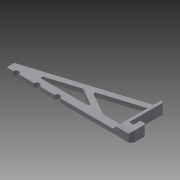
# Autodesk Inventor part: SpoolHandle2
Saved by Autodesk Inventor 2014 (Build 180170000, 170)
## iProperties
Created: 2014-04-03
Part Number: SpoolHandle2
Material: Generic
Document SubType Name: Modeling
Designer: Krzysiek
Density: 1 g/cm^3
Appearance: Default
Author: Krzysiek
Autodesk Inventor part; units mm, degrees
ref_plane "YZ Plane" through (0, 0, 0) normal (1, 0, 0) x (0, 1, 0)
ref_plane "XZ Plane" through (0, 0, 0) normal (0, 1, 0) x (-1, 0, 0)
ref_plane "XY Plane" through (0, 0, 0) normal (0, 0, 1) x (1, 0, 0)
sketch "Sketch1" plane through (0, 0, 0) normal (0, 0, 1) x (1, 0, 0)
  line L0 (0, 0) -> (0, -10)
  line L1 (0, -10) -> (8, -10)
  line L2 (8, -10) -> (8, 11)
  line L3 (-174, 11) -> (-174, 0)
  line L4 (-6.5, -50) -> (-6.5, 0)
  line L5 (-14.5, 0) -> (-14.5, -41.6161)
  line L6 (-80.6593, -20.8766) -> (-44.5, 0)
  line L7 (-44.5, 0) -> (-14.5, 0)
  line L8 (-91.0289, -17.6259) -> (-60.5, 0)
  line L9 (-60.5, 0) -> (-147.2555, 0)
  line L10 (-147.2555, 0) -> (-91.0289, -17.6259)
  line L11 (-6.5, 0) -> (0, 0)
  line L12 (-80.6593, -20.8766) -> (-14.5, -41.6161)
  arc A0 (-164, 11) -> (-156, 11) centre (-160, 11) ccw
  arc A1 (-134, 11) -> (-126, 11) centre (-130, 11) ccw
  arc A2 (-104, 11) -> (-96, 11) centre (-100, 11) ccw
  line L13 (-164, 11) -> (-174, 11)
  line L14 (-134, 11) -> (-156, 11)
  line L15 (8, 11) -> (-96, 11)
  line L16 (-104, 11) -> (-126, 11)
  line L17 (-174, 0) -> (-14.5, -50)
  line L18 (-14.5, -50) -> (-6.5, -50)
  line L19 (-164, 11) -> (-96, 11) construction
  dimension "d0" = 8
  dimension "d1" = 10
  dimension "d2" = 6.5
  dimension "d3" = 182
  dimension "d4" = 11
  dimension "d6" = 8
  dimension "d7" = 50
  dimension "d8" = 30
  dimension "d10" = 8
  dimension "d11" = 30
  dimension "d12" = 8
  dimension "d13" = 160
  dimension "d14" = 30
  dimension "d15" = 30
  dimension "d16" = 8
  dimension "d17" = 8
  constraints: 40 end point, 11 parallel, 7 collinear, 6 point on circle, 3 centre point, 2 equal radius, 2 horizontal, 2 perpendicular, 2 point on line, 1 horizontal alignment, 1 midpoint, 1 vertical
  measures "d0" distance of L0.end L1.end
  measures "d1" distance of L0.start L0.end
  measures "d2" distance of L4.end L0.start
  measures "d3" distance of L2.end L3.start
  measures "d4" distance of L3.start L3.end
  measures "d6" distance between parallel lines of L4 L5
  measures "d7" distance of L4.start L4.end
  measures "d8" distance of L6.end L5.start
  measures "d10" distance between parallel lines of L6 L8
  measures "d11" angle of L8 L9
  measures "d12" diameter of A0
  measures "d13" horizontal distance of A0.centre L0.start
  measures "d14" distance of A1.centre A0.centre
  measures "d15" distance of A2.centre A1.centre
  measures "d16" distance between parallel lines of L17 L12
  measures "d17" distance of L17.end L4.start
extrude "Extrusion1" add sketch "Sketch1" along normal blind 15
sketch "Sketch2" plane through (0, 0, 15) normal (0, 0, 1) x (1, 0, 0)
  line L0 (-174.5, 11) -> (-14.5, 11)
  line L1 (-14.5, 11) -> (-14.5, -59)
  line L2 (-14.5, -59) -> (-174.5, -59)
  line L3 (-174.5, -59) -> (-174.5, 11)
  line L4 (-6.5, 0) -> (0, 0) projected
  line L5 (-14.5, 0) -> (-14.5, -41.6161) projected
  line L6 (8, 11) -> (-96, 11) projected
  dimension "d20" = 70
  dimension "d21" = 160
  constraints: 8 end point, 2 collinear, 2 parallel, 1 horizontal, 1 perpendicular
  measures "d20" distance of L0.end L1.end
  measures "d21" distance of L0.start L0.end
extrude "Extrusion2" cut sketch "Sketch2" against normal blind 9
chamfer "Chamfer1" distance 4 angle 45 1 edges at (8, 11, 7.5)
chamfer "Chamfer2" distance 4 angle 45 1 edges at (-5.25, 11, 15)
chamfer "Chamfer3" distance 2 angle 45 1 edges at (8, -10, 7.5)
chamfer "Chamfer4" distance 4 angle 45 1 edges at (-14.5, -21.5, 15)
chamfer "Chamfer5" distance 5 angle 45 2 edges at (-14.5, -45.8081, 6) (-14.5, 5.5, 6)
fillet "Fillet1" radius 2 1 edges at (-147.2555, 0, 3)
fillet "Fillet2" radius 2 8 edges at (-80.6593, -20.8766, 3) (-44.5, 0, 3) (-60.5, 0, 3) (-91.0289, -17.6259, 3) (-14.5, 0, 8.5) (-14.5, 0, 3) (-14.5, -41.6161, 8.5) (-14.5, -41.6161, 3)
chamfer "Chamfer10" distance 1 angle 45 1 edges at (-6.5, -50, 7.5)
chamfer "Chamfer11" distance 1 angle 45 1 edges at (0, -10, 7.5)
chamfer "Chamfer12" distance 1 angle 45 2 edges at (-174, 0, 3) (-174, 11, 3)
mirror "Mirror1" about plane through (8, 11, 0) normal (0, 1, 0) remove original yes
body "Solid1"
